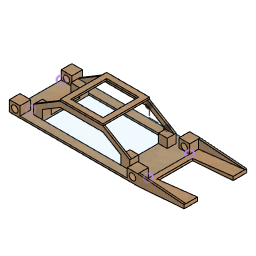
Initial design - Wood Frame v7 (Autodesk Fusion 360 design; units mm, degrees)
Autodesk Fusion 360 part; units mm, degrees
sketch "Sketch1" plane through (0, 0, 0) normal (0, 0, 1) x (1, 0, 0)
  line L0 (360, 175) -> (-360, 175)
  line L1 (-360, 175) -> (-360, -175)
  line L2 (-360, -175) -> (360, -175)
  line L3 (360, -175) -> (360, 175)
  line L4 (360, 175) -> (-360, -175) construction
  line L5 (-360, 175) -> (360, -175) construction
  line L6 (330, 150) -> (308.5714, 150) construction
  line L7 (-308.5714, 150) -> (-330, 150) construction
  line L8 (-330, -150) -> (-308.5714, -150) construction
  line L9 (308.5714, -150) -> (330, -150) construction
  dimension "d1" = 720
  dimension "d2" = 350
  dimension "d7" = 660
  dimension "d8" = 300
  constraint horizontal L0
  constraint perpendicular L0 L1
  constraint parallel L0 L2
  constraint parallel L1 L3
  constraint coincident L4 origin
  constraint coincident L5 origin
  constraint horizontal L6
  constraint parallel L6 L8
  constraint coincident L4 L6.end
  constraint coincident L5 L7.start
  constraint collinear L6 L7
  constraint coincident L4 L8.end
  constraint coincident L5 L9.start
  constraint collinear L8 L9
  measures "d1" distance of L1.end L2.end
  measures "d2" distance of L0.end L1.end
  measures "d7" distance of L8.start L9.end
  measures "d8" distance of L7.end L8.start
extrude "Extrude1" add sketch "Sketch1" along normal blind 10 makes body 1
sketch "Sketch2" plane through (0, 0, 10) normal (0, 0, 1) x (-1, 0, 0)
  line L0 (-360, 175) -> (-360, -175)
  line L1 (-360, -175) -> (360, -175)
  line L2 (360, -175) -> (360, 175)
  line L3 (360, 175) -> (-360, 175)
  line L4 (220, -130) -> (-220, -130)
  line L5 (-220, -130) -> (-220, 130)
  line L6 (-220, 130) -> (220, 130)
  line L7 (220, 130) -> (220, -130)
  line L8 (220, -130) -> (-220, 130) construction
  line L9 (-220, -130) -> (220, 130) construction
  constraint horizontal L4
  constraint perpendicular L4 L5
  constraint parallel L4 L6
  constraint parallel L5 L7
  constraint coincident L8 origin
  constraint coincident L9 origin
extrude "Extrude2" cut sketch "Sketch2" against normal blind 30 contours L4 L5 L6 L7 bodies 1
sketch "Sketch3" plane through (0, 0, 10) normal (0, 0, 1) x (-1, 0, 0)
  line L0 (-220, -130) -> (-220, 130)
  line L1 (-220, 130) -> (220, 130)
  line L2 (220, 130) -> (220, -130)
  line L3 (220, -130) -> (-220, -130)
  line L4 (-360, 175) -> (-360, -175)
  line L5 (-360, -175) -> (360, -175)
  line L6 (360, -175) -> (360, 175)
  line L7 (360, 175) -> (-360, 175)
  line L8 (0, 0) -> (330, 0) construction
  line L9 (330, 0) -> (330, -70) construction
  line L10 (330, -70) -> (330, -175) construction
  line L11 (330, 0) -> (330, 175) construction
  line L12 (0, 0) -> (-330, 0) construction
  line L13 (-330, 0) -> (-330, 175) construction
  line L14 (-330, 0) -> (-330, -175) construction
  line L15 (360, 115.5) -> (300.3842, 115.5)
  line L16 (300.3842, 115.5) -> (300.3842, 175)
  line L17 (300.3842, 175) -> (360, 175)
  line L18 (360, 175) -> (360, 115.5)
  dimension "d9" = 330
  dimension "d10" = 330
  dimension "d33" = 59.5
  constraint coincident L8.start L12.start
  constraint perpendicular L2 L8
  constraint perpendicular L8 L9
  constraint coincident L5 L10.end
  constraint perpendicular L5 L10
  constraint coincident L7 L11.end
  constraint perpendicular L7 L11
  constraint perpendicular L0 L12
  constraint coincident L7 L13.end
  constraint perpendicular L7 L13
  constraint coincident L5 L14.end
  constraint perpendicular L5 L14
  constraint horizontal L15
  constraint vertical L16
  constraint horizontal L17
  constraint vertical L18
  constraint coincident L7 L16.end
  measures "d9" distance of L8.start L8.end
  measures "d10" distance of L8.start L12.end
  measures "d33" distance of L15 L17
extrude "Extrude3" add sketch "Sketch3" along normal blind 50 contours L6 L7 L15 L16 L17 L18 bodies 1
ref_plane "WorkPlane1" through (0, 0, 0) normal (0, 1, 0) x (0, 0, 1)
ref_plane "WorkPlane2" through (0, 0, 0) normal (1, 0, 0) x (0, 1, 0)
mirror "Mirror1" about plane through (0, 0, 0) normal (1, 0, 0) of "Extrude3"
mirror "Mirror2" about plane through (0, 0, 0) normal (0, 1, 0) of "Extrude3", "Mirror1"
sketch "Sketch4" plane through (0, -175, 0) normal (0, -1, 0) x (1, 0, 0)
  line L0 (-360, 60) -> (-360, 0)
  line L1 (-360, 0) -> (360, 0)
  line L2 (360, 0) -> (360, 60)
  line L3 (300.3842, 60) -> (300.3842, 10)
  line L4 (300.3842, 10) -> (-300.3842, 10)
  line L5 (-300.3842, 10) -> (-300.3842, 60)
  circle A0 centre (-330, 30) radius 18.5
  line L6 (360, 60) -> (300.3842, 60)
  line L7 (-300.3842, 60) -> (-360, 60)
  dimension "d21" = 37
  measures "d21" diameter of A0
extrude "Extrude4" cut sketch "Sketch4" against normal blind 26.5 contours A0 bodies 1
sketch "Sketch5" plane through (0, 0, 10) normal (0, 0, 1) x (-1, 0, 0)
  line L0 (-300.3842, -115.5) -> (-300.3842, -175)
  line L1 (-300.3842, -175) -> (300.3842, -175)
  line L2 (300.3842, -175) -> (300.3842, -115.5)
  line L3 (300.3842, -115.5) -> (360, -115.5)
  line L4 (360, -115.5) -> (360, 115.5)
  line L5 (360, 115.5) -> (300.3842, 115.5)
  line L6 (300.3842, 115.5) -> (300.3842, 175)
  line L7 (300.3842, 175) -> (-300.3842, 175)
  line L8 (-300.3842, 175) -> (-300.3842, 115.5)
  line L9 (-300.3842, 115.5) -> (-360, 115.5)
  line L10 (-360, 115.5) -> (-360, -115.5)
  line L11 (-360, -115.5) -> (-300.3842, -115.5)
  line L12 (-220, -130) -> (-220, 130)
  line L13 (-220, 130) -> (220, 130)
  line L14 (220, 130) -> (220, -130)
  line L15 (220, -130) -> (-220, -130)
sketch "Sketch6" plane through (0, -148.5, 0) normal (0, -1, 0) x (1, 0, 0)
  circle A0 centre (-330, 30) radius 18.5
  circle A1 centre (-330, 30) radius 17.75
  dimension "d30" = 35.5
  constraint concentric A0 A1
  measures "d30" diameter of A1
extrude "Extrude5" cut sketch "Sketch6" against normal blind 33 contours A1 bodies 1
mirror "Mirror6" about plane through (0, 0, 0) normal (0, 1, 0) of "Extrude4", "Extrude5"
mirror "Mirror7" about plane through (0, 0, 0) normal (1, 0, 0) of "Extrude4", "Extrude5"
mirror "Mirror8" about plane through (0, 0, 0) normal (0, 1, 0) of "Mirror7"
sketch "Sketch7" plane through (0, 175, 0) normal (0, 1, 0) x (-1, 0, 0)
  circle A0 centre (-330, 30) radius 18.5
  circle A1 centre (330, 30) radius 18.5
  line L0 (-360, 0) -> (360, 0)
  line L1 (360, 0) -> (360, 60)
  line L2 (360, 60) -> (300.3842, 60)
  line L3 (300.3842, 60) -> (300.3842, 10)
  line L4 (300.3842, 10) -> (-300.3842, 10)
  line L5 (-300.3842, 10) -> (-300.3842, 60)
  line L6 (-300.3842, 60) -> (-360, 60)
  line L7 (-360, 60) -> (-360, 0)
  line L8 (-360, 60) -> (-620, 40)
  line L9 (-620, 40) -> (-620, 20)
  line L10 (-620, 20) -> (-360, 0)
  constraint coincident L6.end L7.start
  constraint perpendicular L6 L9
  constraint coincident L0.start L7.end
extrude "Extrude6" add sketch "Sketch7" against normal blind 10 contours L7 L8 L9 L10 bodies 1
mirror "Mirror9" about plane through (0, 0, 0) normal (0, 1, 0) of "Extrude6"
sketch "Sketch8" plane through (0, 175, 0) normal (0, 1, 0) x (-1, 0, 0)
  circle A0 centre (-330, 30) radius 18.5
  circle A1 centre (330, 30) radius 18.5
  line L0 (-360, 0) -> (360, 0)
  line L1 (360, 0) -> (360, 60)
  line L2 (360, 60) -> (300.3842, 60)
  line L3 (300.3842, 60) -> (300.3842, 10)
  line L4 (300.3842, 10) -> (-300.3842, 10)
  line L5 (-300.3842, 10) -> (-300.3842, 60)
  line L6 (-300.3842, 60) -> (-360, 60)
  line L7 (-360, 60) -> (-620, 40)
  line L8 (-620, 40) -> (-620, 20)
  line L9 (-620, 20) -> (-360, 0)
sketch "Sketch9" plane through (0, -165, 0) normal (0, 1, 0) x (-1, 0, 0)
  line L0 (-360, 60) -> (-620, 40)
  line L1 (-620, 40) -> (-620, 20)
  line L2 (-620, 20) -> (-360, 0)
  line L3 (-360, 0) -> (-360, 60)
  line L4 (-620, 40) -> (-360, 10)
  line L5 (-360, 10) -> (-360, 0)
  line L6 (-360, 0) -> (-620, 20)
  line L7 (-620, 20) -> (-620, 40)
  line L8 (-360, 10) -> (-360, 0)
  constraint coincident L0.end L1.start
  constraint coincident L3 L4.end
  constraint coincident L2.end L3.start
  constraint parallel L3 L5
  constraint coincident L1.end L2.start
  constraint parallel L5 L8
extrude "Extrude7" add sketch "Sketch9" along normal blind 330 contours L1 L2 L3 L4 L5 L6 L7 L8 bodies 1
sketch "Sketch10" plane through (3.5912, 0, -31.1241) normal (-0.114624, 0, 0.993409) x (0, -1, 0)
  line L0 (165, 358.7735) -> (165, 620.4985)
  line L1 (165, 620.4985) -> (-165, 620.4985)
  line L2 (-165, 620.4985) -> (-165, 358.7735)
  line L3 (-165, 358.7735) -> (-115.5, 358.7735)
  line L4 (-115.5, 358.7735) -> (115.5, 358.7735)
  line L5 (115.5, 358.7735) -> (165, 358.7735)
  line L6 (100.3889, 620.4985) -> (-99.6111, 620.4985)
  line L7 (-99.6111, 620.4985) -> (-99.6111, 390.4985)
  line L8 (-99.6111, 390.4985) -> (100.3889, 390.4985)
  line L9 (100.3889, 390.4985) -> (100.3889, 620.4985)
  dimension "d46" = 200
  dimension "d49" = 230
  constraint horizontal L6
  constraint vertical L7
  constraint horizontal L8
  constraint vertical L9
  constraint coincident L1 L6.start
  measures "d46" distance of L6.start L6.end
  measures "d49" distance of L6 L8
extrude "Extrude8" cut sketch "Sketch10" against normal blind 70 contours L1 L6 L7 L8 L9 bodies 1
sketch "Sketch11" plane through (0, 0, 10) normal (0, 0, 1) x (-1, 0, 0)
  line L0 (-220, 130) -> (-270, 130)
  line L1 (-270, 130) -> (-270, 80)
  line L2 (-270, 80) -> (-220, 80)
  line L3 (-220, 80) -> (-220, 130)
  line L4 (220, 130) -> (270, 130)
  line L5 (270, 130) -> (270, 80)
  line L6 (270, 80) -> (220, 80)
  line L7 (220, 80) -> (220, 130)
  line L8 (220, -130) -> (270, -130)
  line L9 (270, -130) -> (270, -80)
  line L10 (270, -80) -> (220, -80)
  line L11 (220, -80) -> (220, -130)
  line L12 (-220, -130) -> (-270, -130)
  line L13 (-270, -130) -> (-270, -80)
  line L14 (-270, -80) -> (-220, -80)
  line L15 (-220, -80) -> (-220, -130)
  constraint horizontal L0
  constraint vertical L1
  constraint horizontal L2
  constraint vertical L3
  constraint horizontal L4
  constraint vertical L5
  constraint horizontal L6
  constraint vertical L7
  constraint horizontal L8
  constraint vertical L9
  constraint horizontal L10
  constraint vertical L11
  constraint horizontal L12
  constraint vertical L13
  constraint horizontal L14
  constraint vertical L15
extrude "Extrude9" add sketch "Sketch11" along normal blind 50 bodies 1
sketch "Sketch12" plane through (0, 130, 0) normal (0, 1, 0) x (-1, 0, 0)
  line L0 (-270, 10) -> (-220, 10)
  line L1 (-220, 10) -> (-220, 60)
  line L2 (-220, 60) -> (-270, 60)
  line L3 (-270, 60) -> (-270, 10)
  line L4 (-270, 60) -> (-119.9387, 150.0368)
  line L5 (-119.9387, 150.0368) -> (120.0613, 150.0368)
  line L6 (120.0613, 150.0368) -> (270, 60)
  line L7 (270, 60) -> (220, 60)
  line L8 (220, 60) -> (120.0613, 120.0122)
  line L9 (120.0613, 120.0122) -> (-120, 120.0122)
  line L10 (-120, 120.0122) -> (-220, 60)
  dimension "d52" = 175
  dimension "d53" = 240
  constraint coincident L2.end L3.start
  constraint perpendicular L3 L5
  constraint parallel L2 L7
  constraint parallel L6 L8
  constraint parallel L2 L9
  constraint coincident L1.end L2.start
  measures "d52" distance of L2.end L4.end
  measures "d53" distance of L4.end L5.end
extrude "Extrude10" add sketch "Sketch12" against normal blind 10 contours L2 L4 L5 L6 L7 L8 L9 L10 bodies 1
mirror "Mirror10" about plane through (0, 0, 0) normal (0, 1, 0) of "Extrude10"
sketch "Sketch13" plane through (0, 0, 150.0368) normal (0, 0, 1) x (-1, 0, 0)
  line L0 (120.0613, 130) -> (-119.9387, 130)
  line L1 (-119.9387, 130) -> (-119.9387, 120)
  line L2 (-119.9387, 120) -> (120.0613, 120)
  line L3 (120.0613, 120) -> (120.0613, 130)
  line L4 (-119.9387, 130) -> (120, 130)
  line L5 (120, 130) -> (120, -130)
  line L6 (120, -130) -> (-119.9387, -130)
  line L7 (-119.9387, -130) -> (-119.9387, 130)
  line L8 (-90, 100) -> (90, 100)
  line L9 (90, 100) -> (90, -100)
  line L10 (90, -100) -> (-90, -100)
  line L11 (-90, -100) -> (-90, 100)
  constraint horizontal L4
  constraint vertical L5
  constraint horizontal L6
  constraint vertical L7
  constraint coincident L0.end L1.start
  constraint horizontal L8
  constraint vertical L9
  constraint horizontal L10
  constraint vertical L11
extrude "Extrude11" add sketch "Sketch13" along normal blind 10 separate body contours L0 L1 L2 L4 L5 L7 | L2 L5 L6 L7 makes body 2
sketch "Sketch14" plane through (0, 130, 0) normal (0, 1, 0) x (-1, 0, 0)
  line L0 (220, 10) -> (270, 10)
  line L1 (270, 10) -> (270, 60)
  line L2 (270, 60) -> (120.0613, 150.0368)
  line L3 (120.0613, 150.0368) -> (-119.9387, 150.0368)
  line L4 (-119.9387, 150.0368) -> (-270, 60)
  line L5 (-270, 60) -> (-270, 10)
  line L6 (-270, 10) -> (-220, 10)
  line L7 (-220, 10) -> (-220, 60)
  line L8 (-220, 60) -> (-120, 120.0122)
  line L9 (-120, 120.0122) -> (120.0613, 120.0122)
  line L10 (120.0613, 120.0122) -> (220, 60)
  line L11 (220, 60) -> (220, 10)
  line L12 (-120, 120.0122) -> (-120, 60) construction
  line L13 (-120, 60) -> (-220, 60) construction
  constraint coincident L8.end L9.start
  constraint perpendicular L9 L12
  constraint coincident L7.end L8.start
  constraint perpendicular L7 L13
